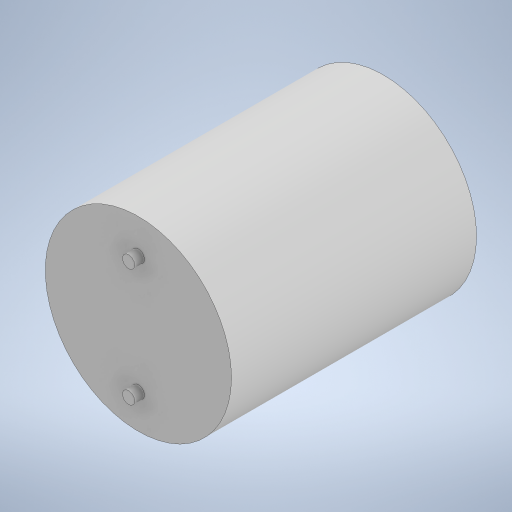
# Autodesk Inventor part: motor
Saved by Autodesk Inventor 2023 (Build 270158000, 158)
## iProperties
Created: 2023-04-09
Part Number: motor
Material: Generic
Document SubType Name: Modeling
Designer: Nikhil
Density: 1 g/cm^3
Appearance: Default
Author: Nikhil
Autodesk Inventor part; units mm, degrees
ref_plane "YZ Plane" through (0, 0, 0) normal (1, 0, 0) x (0, 1, 0)
ref_plane "XZ Plane" through (0, 0, 0) normal (0, 1, 0) x (-1, 0, 0)
ref_plane "XY Plane" through (0, 0, 0) normal (0, 0, 1) x (1, 0, 0)
sketch "Sketch1" plane through (0, 0, 0) normal (0, 0, 1) x (1, 0, 0)
  circle A0 centre (0, 0) radius 19
  dimension "d1" = 38
  constraints: 1 centre point, 1 coincident
  measures "d1" diameter of A0
extrude "Extrusion1" add sketch "Sketch1" along normal blind 50
sketch "Sketch2" plane through (0, 0, 50) normal (0, 0, 1) x (1, 0, 0)
  circle A0 centre (0, 12) radius 1.25
  circle A1 centre (0, -12) radius 1.25
  point P0 (0, 0)
  dimension "d4" = 12
  dimension "d5" = 12
  dimension "d6" = 2.5
  dimension "d7" = 2.5
  constraints: 2 centre point, 2 coincident
  measures "d4" distance of point (0, 0) point (0, 12)
  measures "d5" distance of point (0, 0) point (0, -12)
  measures "d6" diameter of A0
  measures "d7" diameter of A1
extrude "Extrusion2" add sketch "Sketch2" along normal blind 2 contours A0
sketch "Sketch3" plane through (0, 0, 50) normal (0, 0, 1) x (1, 0, 0)
  circle A0 centre (0, -12) radius 1.25
  point P0 (0, 0)
  dimension "d10" = 12
  dimension "d11" = 2.5
  constraints: 1 centre point, 1 coincident
  measures "d10" distance of point (0, 0) point (0, -12)
  measures "d11" diameter of A0
extrude "Extrusion3" add sketch "Sketch3" along normal blind 2
body "Solid1"
